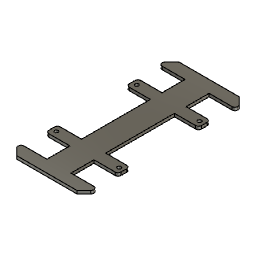
Car_assembly v3 (Autodesk Fusion 360 archive; units mm, degrees)
design "chassis"
Autodesk Fusion 360 part; units mm, degrees
sketch "Sketch1" plane through (0, 0, 0) normal (0, 0, 1) x (1, 0, 0)
  line L0 (0, 50) -> (-50, 50)
  line L1 (-50, 50) -> (-61.4645, 38.5355)
  line L2 (-57.9289, 30) -> (-20, 30)
  line L3 (-20, 30) -> (-20, -8.2114)
  line L4 (-20, -8.2114) -> (-55.1, -8.2114)
  line L5 (-60, -13.1114) -> (-60, -22.6237)
  line L6 (-55.1, -27.5237) -> (-20, -27.5237)
  line L7 (-20, -27.5237) -> (-20, -84.6544)
  line L8 (50, 50) -> (61.4645, 38.5355)
  line L9 (20, -27.5237) -> (20, -84.6544)
  line L10 (20, 30) -> (20, -8.2114)
  line L11 (0, 50) -> (50, 50)
  line L12 (55.1, -27.5237) -> (20, -27.5237)
  line L13 (60, -13.1114) -> (60, -22.6237)
  line L14 (20, -8.2114) -> (55.1, -8.2114)
  line L15 (57.9289, 30) -> (20, 30)
  arc A0 (-61.4645, 38.5355) -> (-57.9289, 30) centre (-57.9289, 35) ccw
  arc A1 (57.9289, 30) -> (61.4645, 38.5355) centre (57.9289, 35) ccw
  arc A2 (-55.1, -8.2114) -> (-60, -13.1114) centre (-55.1, -13.1114) ccw
  arc A3 (-60, -22.6237) -> (-55.1, -27.5237) centre (-55.1, -22.6237) ccw
  arc A4 (60, -13.1114) -> (55.1, -8.2114) centre (55.1, -13.1114) ccw
  arc A5 (55.1, -27.5237) -> (60, -22.6237) centre (55.1, -22.6237) ccw
  circle A6 centre (52.0901, -17.8676) radius 3
  circle A7 centre (-52.0901, -17.8676) radius 3
  line L16 (-50, -219.3089) -> (-61.4645, -207.8444)
  line L17 (55.1, -141.7852) -> (20, -141.7852)
  line L18 (20, -141.7852) -> (20, -84.6544)
  line L19 (0, -219.3089) -> (-50, -219.3089)
  line L20 (20, -199.3089) -> (20, -161.0975)
  line L21 (-57.9289, -199.3089) -> (-20, -199.3089)
  arc A8 (-57.9289, -199.3089) -> (-61.4645, -207.8444) centre (-57.9289, -204.3089) ccw
  line L22 (-20, -141.7852) -> (-20, -84.6544)
  circle A9 centre (52.0901, -151.4413) radius 3
  arc A10 (-55.1, -141.7852) -> (-60, -146.6852) centre (-55.1, -146.6852) ccw
  line L23 (-55.1, -141.7852) -> (-20, -141.7852)
  line L24 (-20, -161.0975) -> (-55.1, -161.0975)
  line L25 (60, -156.1975) -> (60, -146.6852)
  arc A11 (-60, -156.1975) -> (-55.1, -161.0975) centre (-55.1, -156.1975) ccw
  line L26 (0, -219.3089) -> (50, -219.3089)
  arc A12 (55.1, -161.0975) -> (60, -156.1975) centre (55.1, -156.1975) ccw
  line L27 (-20, -199.3089) -> (-20, -161.0975)
  line L28 (20, -161.0975) -> (55.1, -161.0975)
  line L29 (-60, -156.1975) -> (-60, -146.6852)
  arc A13 (61.4645, -207.8444) -> (57.9289, -199.3089) centre (57.9289, -204.3089) ccw
  circle A14 centre (-52.0901, -151.4413) radius 3
  line L30 (50, -219.3089) -> (61.4645, -207.8444)
  line L31 (57.9289, -199.3089) -> (20, -199.3089)
  arc A15 (60, -146.6852) -> (55.1, -141.7852) centre (55.1, -146.6852) ccw
  point P0 (0, -169.3089)
  dimension "d1" = 5
  dimension "d2" = 5
  dimension "d3" = 4.9
  dimension "d4" = 6
  constraint horizontal L0
  constraint parallel L0 L2
  constraint perpendicular L2 L3
  constraint perpendicular L3 L4
  constraint perpendicular L4 L5
  constraint perpendicular L5 L6
  constraint perpendicular L6 L7
  constraint tangent L1 A0
  constraint tangent L2 A0
  constraint tangent L8 A1
  constraint tangent L15 A1
  constraint tangent L4 A2
  constraint tangent L5 A2
  constraint tangent L5 A3
  constraint tangent L6 A3
  constraint equal A2 A3
  constraint tangent L13 A4
  constraint tangent L14 A4
  constraint equal A2 A4
  constraint tangent L12 A5
  constraint tangent L13 A5
  constraint equal A2 A5
  measures "d1" radius of A0
  measures "d2" radius of A1
  measures "d3" radius of A2
  measures "d4" diameter of A6
extrude "Extrude1" add sketch "Sketch1" along normal blind 10
extrude "Extrude2" cut 1 faces at (6.6667, -65.6109, 10) along direction (0, 0, -1) blind 5

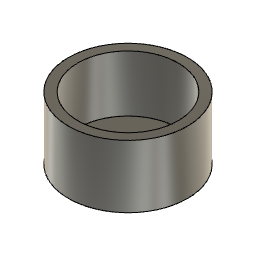
design "wheel"
Autodesk Fusion 360 part; units mm, degrees
sketch "Sketch1" plane through (0, 0, 0) normal (0, 0, 1) x (1, 0, 0)
  circle A0 centre (0, 0) radius 47.5
  dimension "d7" = 95
  constraint coincident A0.centre origin
  measures "d7" diameter of A0
extrude "Extrude1" add sketch "Sketch1" along normal blind 50
sketch "Sketch3" plane through (0, 0, 50) normal (0, 0, 1) x (-1, 0, 0)
  circle A0 centre (0, 0) radius 47.5
  circle A1 centre (0, 0) radius 40
  dimension "d3" = 80
  dimension "d4" = 144.2221
  constraint coincident A0.centre A1.centre
  measures "d3" diameter of A1
extrude "Extrude2" cut sketch "Sketch3" against normal blind 45 contours A1

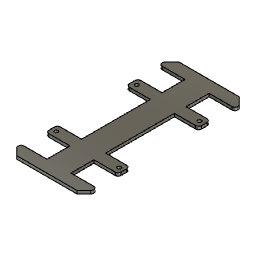
design "chassis"
Autodesk Fusion 360 part; units mm, degrees
sketch "Sketch1" plane through (0, 0, 0) normal (0, 0, 1) x (1, 0, 0)
  line L0 (0, 50) -> (-50, 50)
  line L1 (-50, 50) -> (-61.4645, 38.5355)
  line L2 (-57.9289, 30) -> (-20, 30)
  line L3 (-20, 30) -> (-20, -8.2114)
  line L4 (-20, -8.2114) -> (-55.1, -8.2114)
  line L5 (-60, -13.1114) -> (-60, -22.6237)
  line L6 (-55.1, -27.5237) -> (-20, -27.5237)
  line L7 (-20, -27.5237) -> (-20, -84.6544)
  line L8 (50, 50) -> (61.4645, 38.5355)
  line L9 (20, -27.5237) -> (20, -84.6544)
  line L10 (20, 30) -> (20, -8.2114)
  line L11 (0, 50) -> (50, 50)
  line L12 (55.1, -27.5237) -> (20, -27.5237)
  line L13 (60, -13.1114) -> (60, -22.6237)
  line L14 (20, -8.2114) -> (55.1, -8.2114)
  line L15 (57.9289, 30) -> (20, 30)
  arc A0 (-61.4645, 38.5355) -> (-57.9289, 30) centre (-57.9289, 35) ccw
  arc A1 (57.9289, 30) -> (61.4645, 38.5355) centre (57.9289, 35) ccw
  arc A2 (-55.1, -8.2114) -> (-60, -13.1114) centre (-55.1, -13.1114) ccw
  arc A3 (-60, -22.6237) -> (-55.1, -27.5237) centre (-55.1, -22.6237) ccw
  arc A4 (60, -13.1114) -> (55.1, -8.2114) centre (55.1, -13.1114) ccw
  arc A5 (55.1, -27.5237) -> (60, -22.6237) centre (55.1, -22.6237) ccw
  circle A6 centre (52.0901, -17.8676) radius 3
  circle A7 centre (-52.0901, -17.8676) radius 3
  line L16 (-50, -219.3089) -> (-61.4645, -207.8444)
  line L17 (55.1, -141.7852) -> (20, -141.7852)
  line L18 (20, -141.7852) -> (20, -84.6544)
  line L19 (0, -219.3089) -> (-50, -219.3089)
  line L20 (20, -199.3089) -> (20, -161.0975)
  line L21 (-57.9289, -199.3089) -> (-20, -199.3089)
  arc A8 (-57.9289, -199.3089) -> (-61.4645, -207.8444) centre (-57.9289, -204.3089) ccw
  line L22 (-20, -141.7852) -> (-20, -84.6544)
  circle A9 centre (52.0901, -151.4413) radius 3
  arc A10 (-55.1, -141.7852) -> (-60, -146.6852) centre (-55.1, -146.6852) ccw
  line L23 (-55.1, -141.7852) -> (-20, -141.7852)
  line L24 (-20, -161.0975) -> (-55.1, -161.0975)
  line L25 (60, -156.1975) -> (60, -146.6852)
  arc A11 (-60, -156.1975) -> (-55.1, -161.0975) centre (-55.1, -156.1975) ccw
  line L26 (0, -219.3089) -> (50, -219.3089)
  arc A12 (55.1, -161.0975) -> (60, -156.1975) centre (55.1, -156.1975) ccw
  line L27 (-20, -199.3089) -> (-20, -161.0975)
  line L28 (20, -161.0975) -> (55.1, -161.0975)
  line L29 (-60, -156.1975) -> (-60, -146.6852)
  arc A13 (61.4645, -207.8444) -> (57.9289, -199.3089) centre (57.9289, -204.3089) ccw
  circle A14 centre (-52.0901, -151.4413) radius 3
  line L30 (50, -219.3089) -> (61.4645, -207.8444)
  line L31 (57.9289, -199.3089) -> (20, -199.3089)
  arc A15 (60, -146.6852) -> (55.1, -141.7852) centre (55.1, -146.6852) ccw
  point P0 (0, -169.3089)
  dimension "d1" = 5
  dimension "d2" = 5
  dimension "d3" = 4.9
  dimension "d4" = 6
  constraint horizontal L0
  constraint parallel L0 L2
  constraint perpendicular L2 L3
  constraint perpendicular L3 L4
  constraint perpendicular L4 L5
  constraint perpendicular L5 L6
  constraint perpendicular L6 L7
  constraint tangent L1 A0
  constraint tangent L2 A0
  constraint tangent L8 A1
  constraint tangent L15 A1
  constraint tangent L4 A2
  constraint tangent L5 A2
  constraint tangent L5 A3
  constraint tangent L6 A3
  constraint equal A2 A3
  constraint tangent L13 A4
  constraint tangent L14 A4
  constraint equal A2 A4
  constraint tangent L12 A5
  constraint tangent L13 A5
  constraint equal A2 A5
  measures "d1" radius of A0
  measures "d2" radius of A1
  measures "d3" radius of A2
  measures "d4" diameter of A6
extrude "Extrude1" add sketch "Sketch1" along normal blind 10
extrude "Extrude2" cut 1 faces at (6.6667, -65.6109, 10) along direction (0, 0, -1) blind 5
